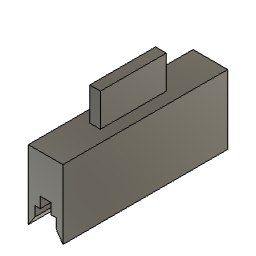
Servo Actuator v3 (Autodesk Fusion 360 design; units mm, degrees)
Autodesk Fusion 360 part; units mm, degrees
sketch "Sketch1" plane through (0, 0, 0) normal (0, 1, 0) x (1, 0, 0) in component "Servo Actuator"
  line L0 (0, 0) -> (3.25, 0)
  line L1 (3.25, 0) -> (3.25, 3)
  line L2 (3.25, 0) -> (5.25, 0)
  line L3 (5.25, 0) -> (5.25, 6)
  line L4 (5.25, 6) -> (3.25, 3)
  line L5 (0, 0) -> (0, -3.25)
  line L6 (0, -3.25) -> (1.625, -3.25)
  line L7 (1.625, -3.25) -> (1.625, 0)
  line L8 (5.25, 0) -> (5.25, -3.25)
  line L9 (5.25, -3.25) -> (1.625, -3.25)
  line L10 (0, -3.25) -> (0, -5.75)
  line L11 (5.25, -3.25) -> (5.25, -5.75)
  line L12 (5.25, -5.75) -> (0, -5.75)
  line L13 (0, -5.75) -> (0, -35)
  line L14 (0, -35) -> (5.25, -35)
  line L15 (5.25, -35) -> (5.25, -5.75)
  line L16 (-5.25, 0) -> (-5.25, -3.25)
  line L17 (0, 0) -> (-3.25, 0)
  line L18 (-5.25, -5.75) -> (0, -5.75)
  line L19 (-5.25, -35) -> (-5.25, -5.75)
  line L20 (-5.25, -3.25) -> (-5.25, -5.75)
  line L21 (-1.625, -3.25) -> (-1.625, 0)
  line L22 (-5.25, 6) -> (-3.25, 3)
  line L23 (-5.25, 0) -> (-5.25, 6)
  line L24 (-3.25, 0) -> (-5.25, 0)
  line L25 (0, -35) -> (-5.25, -35)
  line L26 (0, -3.25) -> (-1.625, -3.25)
  line L27 (-3.25, 0) -> (-3.25, 3)
  line L28 (-5.25, -3.25) -> (-1.625, -3.25)
  dimension "d1" = 3.25
  dimension "d2" = 3
  dimension "d6" = 2
  dimension "d7" = 6
  dimension "d8" = 3.25
  dimension "d9" = 1.625
  dimension "d10" = 3.25
  dimension "d12" = 2.5
  dimension "d13" = 2.5
  dimension "d14" = 29.25
  dimension "d15" = 5.25
  constraint coincident L0.start L5.start
  constraint horizontal L0
  constraint perpendicular L0 L1
  constraint perpendicular L1 L2
  constraint perpendicular L2 L3
  constraint perpendicular L0 L5
  constraint perpendicular L5 L6
  constraint midpoint L0 L7.end
  constraint perpendicular L2 L8
  constraint perpendicular L6 L10
  constraint perpendicular L9 L11
  constraint perpendicular L0 L13
  constraint perpendicular L13 L14
  constraint symmetric L0.start L10 L5.start
  constraint symmetric L0.end L10 L17.end
  constraint symmetric L1.end L10 L22.end
  constraint symmetric L2.end L10 L16.start
  constraint symmetric L3.end L10 L22.start
  constraint symmetric L5.end L10 L6.start
  constraint symmetric L6.end L10 L21.start
  constraint symmetric L7.end L10 L21.end
  constraint symmetric L8.end L10 L16.end
  constraint symmetric L12.end L10 L13.start
  constraint symmetric L10 L11.end L18.start
  constraint symmetric L10 L13.end L14.start
  constraint symmetric L10 L14.end L19.start
  measures "d1" distance of L0.start L0.end
  measures "d2" distance of L0.end L1.end
  measures "d6" distance of L0.end L2.end
  measures "d7" distance of L2.end L3.end
  measures "d8" distance of L0.start L5.end
  measures "d9" distance of L5.end L6.end
  measures "d10" distance of L2.end L8.end
  measures "d12" distance of L5.end L10.end
  measures "d13" distance of L8.end L11.end
  measures "d14" distance of L10.end L13.end
  measures "d15" distance of L13.end L14.end
extrude "Extrude1" add sketch "Sketch1" along normal mid plane 50 contours L0 L2 L7 L8 L9 | L6 L9 L10 L11 L12 | L10 L18 L20 L26 L28 | L16 L17 L21 L24 L28 | L1 L2 L3 L4 | L12 L13 L14 L15 | L13 L18 L19 L25 | L22 L23 L24 L27 makes body 1 in component "Servo Actuator"
extrude "Extrude2" cut 1 faces at (-1.75, -8.3333, 35) along direction (0, 0, -1) blind 20 on bodies 1 bodies 1 in component "Servo Actuator"
extrude "Extrude3" add sketch "Sketch1" along normal mid plane 35 separate body contours L0 L5 L6 L7 | L5 L17 L21 L26 makes body 2 in component "Servo Actuator"
sketch "Sketch2" plane through (0, 0, 0) normal (0, 0, 1) x (1, 0, 0) in component "Servo Actuator"
  line L0 (1.625, -10) -> (-1.625, -10)
  line L1 (-1.625, -10) -> (-1.625, 10)
  line L2 (-1.625, 10) -> (1.625, 10)
  line L3 (1.625, 10) -> (1.625, -10)
  line L4 (1.625, -10) -> (-1.625, 10) construction
  line L5 (-1.625, -10) -> (1.625, 10) construction
  dimension "d30" = 3.25
  dimension "d31" = 20
  constraint horizontal L0
  constraint perpendicular L0 L1
  constraint parallel L0 L2
  constraint parallel L1 L3
  constraint coincident L4 origin
  constraint coincident L5 origin
  measures "d30" distance of L1.end L2.end
  measures "d31" distance of L0.end L1.end
extrude "Extrude4" add sketch "Sketch2" along normal blind 25 bodies 2 in component "Servo Actuator"
extrude "Extrude5" cut sketch "Sketch2" along normal blind 15 bodies 1 in component "Servo Actuator"
component "Servo Actuator" placed x (1, 0, 0) y (0, 1, 0) z (0, 0, 1) at (0, 0, 0)
equation "d9 = ( 3.25 / 2 ) * 1 mm"
equation "d25 = ( 35 / 2 ) * 1 mm"
